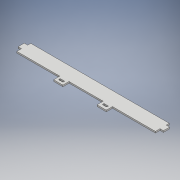
# Autodesk Inventor part: poprz_690
Saved by Autodesk Inventor 2017 (Build 210142000, 142)
## iProperties
Created: 2019-10-27
Part Number: poprz_690
Material: Ogólny
Document SubType Name: Modeling
Designer: patry
Density: 1 g/cm^3
Appearance: Domyślna
Author: patry
Autodesk Inventor part; units mm, degrees
ref_plane "YZ Plane" through (0, 0, 0) normal (1, 0, 0) x (0, 1, 0)
ref_plane "XZ Plane" through (0, 0, 0) normal (0, 1, 0) x (-1, 0, 0)
ref_plane "XY Plane" through (0, 0, 0) normal (0, 0, 1) x (1, 0, 0)
sketch "Szkic1" plane through (0, 0, 0) normal (0, 0, 1) x (1, 0, 0)
  line L0 (-236, 32.5) -> (236, 32.5)
  line L1 (236, 32.5) -> (236, -32.5)
  line L2 (236, -32.5) -> (-236, -32.5)
  line L3 (-236, -32.5) -> (-236, 32.5)
  line L4 (-236, 32.5) -> (236, -32.5) construction
  line L5 (236, 32.5) -> (-236, -32.5) construction
  line L6 (-225, -12.5) -> (225, -12.5)
  line L7 (225, -12.5) -> (225, 32.5)
  line L8 (225, 32.5) -> (-225, 32.5)
  line L9 (-225, 32.5) -> (-225, -12.5)
  line L10 (-225, -12.5) -> (225, 32.5) construction
  line L11 (225, -12.5) -> (-225, 32.5) construction
  line L12 (-236, 22.5) -> (-225, 22.5)
  line L13 (-225, 22.5) -> (-225, 2.5)
  line L14 (-225, 2.5) -> (-236, 2.5)
  line L15 (-236, 2.5) -> (-236, 22.5)
  line L16 (225, 22.5) -> (236, 22.5)
  line L17 (236, 22.5) -> (236, 2.5)
  line L18 (236, 2.5) -> (225, 2.5)
  line L19 (225, 2.5) -> (225, 22.5)
  line L20 (-85.5, -12.5) -> (-55.5, -12.5)
  line L21 (-55.5, -12.5) -> (-55.5, -32.5)
  line L22 (-55.5, -32.5) -> (-85.5, -32.5)
  line L23 (-85.5, -32.5) -> (-85.5, -12.5)
  line L24 (-85.5, -12.5) -> (-55.5, -32.5) construction
  line L25 (-55.5, -12.5) -> (-85.5, -32.5) construction
  line L26 (55.5, -12.5) -> (85.5, -12.5)
  line L27 (85.5, -12.5) -> (85.5, -32.5)
  line L28 (85.5, -32.5) -> (55.5, -32.5)
  line L29 (55.5, -32.5) -> (55.5, -12.5)
  line L30 (55.5, -12.5) -> (85.5, -32.5) construction
  line L31 (85.5, -12.5) -> (55.5, -32.5) construction
  line L32 (-76, -24.5) -> (-65, -24.5)
  line L33 (-63, -22.5) -> (-63, -20.5)
  line L34 (-65, -18.5) -> (-76, -18.5)
  line L35 (-78, -20.5) -> (-78, -22.5)
  line L36 (-78, -24.5) -> (-63, -18.5) construction
  line L37 (-63, -24.5) -> (-78, -18.5) construction
  line L38 (65, -17.5) -> (76, -17.5)
  line L39 (78, -19.5) -> (78, -21.5)
  line L40 (76, -23.5) -> (65, -23.5)
  line L41 (63, -21.5) -> (63, -19.5)
  line L42 (63, -17.5) -> (78, -23.5) construction
  line L43 (78, -17.5) -> (63, -23.5) construction
  arc A0 (-65, -24.5) -> (-63, -22.5) centre (-65, -22.5) ccw
  arc A1 (-63, -20.5) -> (-65, -18.5) centre (-65, -20.5) ccw
  arc A2 (-76, -18.5) -> (-78, -20.5) centre (-76, -20.5) ccw
  arc A3 (-78, -22.5) -> (-76, -24.5) centre (-76, -22.5) ccw
  arc A4 (63, -21.5) -> (65, -23.5) centre (65, -21.5) ccw
  arc A5 (65, -17.5) -> (63, -19.5) centre (65, -19.5) ccw
  arc A6 (78, -19.5) -> (76, -17.5) centre (76, -19.5) ccw
  arc A7 (76, -23.5) -> (78, -21.5) centre (76, -21.5) ccw
  point P0 (0, 0)
  point P1 (0, 0)
  point P2 (-70.5, -22.5)
  point P3 (70.5, -22.5)
  point P4 (-70.5, -21.5)
  point P5 (70.5, -20.5)
  dimension "d0" = 472
  dimension "d1" = 65
  dimension "d2" = 450
  dimension "d3" = 45
  dimension "d4" = 10
  dimension "d5" = 11
  dimension "d6" = 20
  dimension "d7" = 10
  dimension "d8" = 20
  dimension "d9" = 141
  dimension "d10" = 20
  dimension "d11" = 20
  dimension "d12" = 30
  dimension "d13" = 30
  dimension "d15" = 70.5
  dimension "d16" = 15
  dimension "d17" = 6
  dimension "d18" = 6
  dimension "d19" = 15
  dimension "d20" = 6
  dimension "d21" = 5
  dimension "d22" = 2
  constraints: 88 end point, 21 point on line, 16 parallel, 16 point on circle, 16 tangent, 9 midpoint, 8 centre point, 8 horizontal, 8 perpendicular, 7 equal radius, 1 coincident, 1 horizontal alignment
  measures "d0" distance of L1.end L2.end
  measures "d1" distance of L0.end L1.end
  measures "d2" distance of L8.end L7.end
  measures "d3" distance of L7.end L6.end
  measures "d4" distance between parallel lines of L0 L12
  measures "d5" distance between parallel lines of L9 L3
  measures "d6" distance of L16.end L17.end
  measures "d7" distance between parallel lines of L0 L16
  measures "d8" distance between parallel lines of L12 L14
  measures "d9" distance of point (-70.5, -22.5) point (70.5, -22.5)
  measures "d10" distance of L26.end L27.end
  measures "d11" distance of L22.end L20.start
  measures "d12" distance between parallel lines of L23 L21
  measures "d13" distance between parallel lines of L29 L27
  measures "d15" horizontal distance of point (0, 0) point (-70.5, -22.5)
  measures "d16" distance of L37.end L36.end
  measures "d17" distance of L36.end L37.start
  measures "d18" distance between parallel lines of L6 L34
  measures "d19" distance of L42.end L43.end
  measures "d20" distance of L43.start L42.end
  measures "d21" distance between parallel lines of L6 L38
  measures "d22" radius of A0
extrude "Wyciągnięcie proste1" add sketch "Szkic1" along normal blind 5 contours L0 L7 L6 L9 | L12 L9 L14 L3 | L16 L1 L18 L7 | L23 L6 L21 L2 | L27 L2 L29 L6
equation "\"d15\" = 0.5 * d9"
